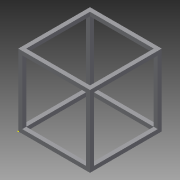
# Autodesk Inventor part: Basic Frame
Saved by Autodesk Inventor 2015 SP1 (Build 190203100, 203)
## iProperties
Created: 2014-10-09
Part Number: Basic Frame
Material: Generic
Document SubType Name: Modeling
Designer: Jordan M
Density: 1 g/cm^3
Appearance: Default
Author: Jordan M
Autodesk Inventor part; units mm, degrees
ref_plane "YZ Plane" through (0, 0, 0) normal (1, 0, 0) x (0, 1, 0)
ref_plane "XZ Plane" through (0, 0, 0) normal (0, 1, 0) x (-1, 0, 0)
ref_plane "XY Plane" through (0, 0, 0) normal (0, 0, 1) x (1, 0, 0)
sketch "Sketch1" plane through (0, 0, 0) normal (0, 1, 0) x (-1, 0, 0)
  line L0 (0, 0) -> (-457.2, 0)
  line L1 (-457.2, 0) -> (-457.2, -25.4)
  line L2 (-457.2, -25.4) -> (0, -25.4)
  line L3 (0, -25.4) -> (0, 0)
  line L4 (0, 0) -> (-25.4, 0)
  line L5 (-25.4, 0) -> (-25.4, -457.2)
  line L6 (-25.4, -457.2) -> (0, -457.2)
  line L7 (0, -457.2) -> (0, 0)
  line L8 (0, -457.2) -> (-457.2, -457.2)
  line L9 (-457.2, -457.2) -> (-457.2, -431.8)
  line L10 (-457.2, -431.8) -> (0, -431.8)
  line L11 (0, -431.8) -> (0, -457.2)
  line L12 (-457.2, 0) -> (-431.8, 0)
  line L13 (-431.8, 0) -> (-431.8, -457.2)
  line L14 (-431.8, -457.2) -> (-457.2, -457.2)
  line L15 (-457.2, -457.2) -> (-457.2, 0)
  dimension "d0" = 457.2
  dimension "d1" = 25.4
  dimension "d2" = 25.4
  dimension "d3" = 457.2
  dimension "d4" = 457.2
  dimension "d5" = 25.4
  dimension "d6" = 25.4
  constraints: 32 end point, 8 parallel, 4 horizontal, 4 perpendicular, 1 point on line
  measures "d0" distance of L2.end L1.end
  measures "d1" distance of L1.end L0.end
  measures "d2" distance of L6.end L5.end
  measures "d3" distance of L5.end L4.end
  measures "d4" distance of L9.end L10.end
  measures "d5" distance of L8.end L9.end
  measures "d6" distance of L13.end L14.end
sketch "Sketch2" plane through (0, 0, 0) normal (0, 1, 0) x (-1, 0, 0)
  line L0 (0, 0) -> (-25.4, 0)
  line L1 (-25.4, 0) -> (-25.4, -25.4)
  line L2 (-25.4, -25.4) -> (0, -25.4)
  line L3 (0, -25.4) -> (0, 0)
  line L4 (0, -457.1579) -> (-25.4, -457.1579)
  line L5 (-25.4, -457.1579) -> (-25.4, -431.7579)
  line L6 (-25.4, -431.7579) -> (0, -431.7579)
  line L7 (0, -431.7579) -> (0, -457.1579)
  line L8 (-457.244, -457.1579) -> (-431.844, -457.1579)
  line L9 (-431.844, -457.1579) -> (-431.844, -431.7579)
  line L10 (-431.844, -431.7579) -> (-457.244, -431.7579)
  line L11 (-457.244, -431.7579) -> (-457.244, -457.1579)
  line L12 (-457.244, 0) -> (-431.844, 0)
  line L13 (-431.844, 0) -> (-431.844, -25.4)
  line L14 (-431.844, -25.4) -> (-457.244, -25.4)
  line L15 (-457.244, -25.4) -> (-457.244, 0)
  dimension "d7" = 25.4
  dimension "d8" = 25.4
  dimension "d9" = 25.4
  dimension "d10" = 25.4
  dimension "d11" = 25.4
  dimension "d12" = 25.4
  dimension "d13" = 25.4
  dimension "d14" = 25.4
  constraints: 32 end point, 8 parallel, 4 horizontal, 4 perpendicular
  measures "d7" distance of L2.end L1.end
  measures "d8" distance of L1.end L0.end
  measures "d9" distance of L5.end L6.end
  measures "d10" distance of L4.end L5.end
  measures "d11" distance of L10.end L9.end
  measures "d12" distance of L9.end L8.end
  measures "d13" distance of L13.end L14.end
  measures "d14" distance of L12.end L13.end
sketch "Sketch3" plane through (0, 0, 0) normal (0, 0, 1) x (1, 0, 0)
  point P0 (0, 0)
sketch "Sketch4" plane through (0, 0, 0) normal (0, 0, 1) x (1, 0, 0)
  point P0 (0, 0)
extrude "Extrusion1" add sketch "Sketch1" along normal blind 25.4 contours L3 L2 L5 L0 | L5 L2 L13 L0 | L7 L10 L5 L2 | L13 L2 L1 L0 | L7 L6 L5 L10 | L13 L10 L15 L2 | L5 L8 L13 L10 | L13 L8 L9 L10
extrude "Extrusion2" add sketch "Sketch2" along normal blind 457.2
sketch "Sketch5" plane through (0, 457.2, 0) normal (0, 1, 0) x (1, 0, 0)
  line L0 (0, 0) -> (25.4, 0)
  line L1 (25.4, 0) -> (25.4, 25.4)
  line L2 (25.4, 25.4) -> (0, 25.4)
  line L3 (0, 25.4) -> (0, 0)
  line L4 (0, 457.1579) -> (25.4, 457.1579)
  line L5 (25.4, 457.1579) -> (25.4, -0.0421)
  line L6 (25.4, -0.0421) -> (0, -0.0421)
  line L7 (0, -0.0421) -> (0, 457.1579)
  line L8 (457.244, 25.4) -> (431.844, 25.4) projected
  line L9 (0, 0) -> (457.2, 0)
  line L10 (457.2, 0) -> (457.2, 25.4)
  line L11 (457.2, 25.4) -> (0, 25.4)
  line L12 (0, 25.4) -> (0, 0)
  line L13 (431.844, 431.7579) -> (457.244, 431.7579) projected
  line L14 (0, 457.1579) -> (457.2, 457.1579)
  line L15 (457.2, 457.1579) -> (457.2, 431.7579)
  line L16 (457.2, 431.7579) -> (0, 431.7579)
  line L17 (0, 431.7579) -> (0, 457.1579)
  line L18 (457.244, 0) -> (431.844, 0)
  line L19 (431.844, 0) -> (431.844, 457.2)
  line L20 (431.844, 457.2) -> (457.244, 457.2)
  line L21 (457.244, 457.2) -> (457.244, 0)
  dimension "d19" = 25.4
  dimension "d20" = 457.2
  dimension "d21" = 457.2
  dimension "d22" = 457.2
  dimension "d23" = 25.4
  dimension "d24" = 457.2
  constraints: 40 end point, 10 parallel, 5 horizontal, 5 perpendicular, 2 point on line
  measures "d19" distance of L5.end L6.end
  measures "d20" distance of L4.end L5.end
  measures "d21" distance of L11.end L10.end
  measures "d22" distance of L15.end L16.end
  measures "d23" distance of L19.end L20.end
  measures "d24" distance of L18.end L19.end
extrude "Extrusion3" add sketch "Sketch5" against normal blind 25.4 contours L3 L2 L1 L0 | L0 L5 L6 L7 | L1 L11 L19 L9 | L7 L16 L5 L2 | L19 L8 L10 L9 | L7 L4 L5 L16 | L5 L14 L19 L16 | L19 L13 L21 L8 | L10 L8 L21 L18 | L19 L14 L15 L13 | L19 L20 L21 L13 L15 L14
body "Solid1"
